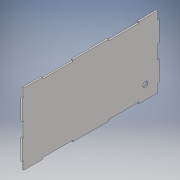
# Autodesk Inventor part: case_side_A
Saved by Autodesk Inventor 2019 (Build 230136000, 136)
## iProperties
Created: 2019-07-12
Part Number: case_side_A
Material: Generic
Document SubType Name: Modeling
Designer: Lino P
Density: 1 g/cm^3
Appearance: Default
Author: Lino P
Autodesk Inventor part; units mm, degrees
ref_plane "YZ Plane" through (0, 0, 0) normal (1, 0, 0) x (0, 1, 0)
ref_plane "XZ Plane" through (0, 0, 0) normal (0, 1, 0) x (-1, 0, 0)
ref_plane "XY Plane" through (0, 0, 0) normal (0, 0, 1) x (1, 0, 0)
sketch "Sketch1" plane through (0, 0, 0) normal (0, 0, 1) x (1, 0, 0)
  line L0 (-15, 60.2) -> (357, 60.2)
  line L1 (357, 60.2) -> (357, -80)
  line L2 (357, -80) -> (-15, -80)
  line L3 (-15, -80) -> (-15, 60.2)
  line L4 (-15, -9.9) -> (357, -9.9) construction
  line L5 (171, 60.2) -> (171, -80) construction
  line L6 (-15, 44.2) -> (-9, 44.2)
  line L7 (-9, 44.2) -> (-9, 4.2)
  line L8 (-9, 4.2) -> (-15, 4.2)
  line L9 (-15, 4.2) -> (-15, 44.2)
  line L10 (-15, -64) -> (-9, -64)
  line L11 (-9, -64) -> (-9, -24)
  line L12 (-9, -24) -> (-15, -24)
  line L13 (-15, -24) -> (-15, -64)
  line L14 (357, 44.2) -> (351, 44.2)
  line L15 (351, 44.2) -> (351, 4.2)
  line L16 (351, 4.2) -> (357, 4.2)
  line L17 (357, 4.2) -> (357, 44.2)
  line L18 (351, -64) -> (351, -24)
  line L19 (357, -64) -> (351, -64)
  line L20 (357, -24) -> (357, -64)
  line L21 (351, -24) -> (357, -24)
  line L22 (25, 60.2) -> (110, 60.2)
  line L23 (110, 60.2) -> (110, 54.2)
  line L24 (110, 54.2) -> (25, 54.2)
  line L25 (25, 54.2) -> (25, 60.2)
  line L26 (317, 60.2) -> (232, 60.2)
  line L27 (232, 60.2) -> (232, 54.2)
  line L28 (232, 54.2) -> (317, 54.2)
  line L29 (317, 54.2) -> (317, 60.2)
  line L30 (25, -80) -> (110, -80)
  line L31 (110, -80) -> (110, -74)
  line L32 (110, -74) -> (25, -74)
  line L33 (25, -74) -> (25, -80)
  line L34 (317, -74) -> (317, -80)
  line L35 (232, -80) -> (232, -74)
  line L36 (232, -74) -> (317, -74)
  line L37 (317, -80) -> (232, -80)
  line L38 (-15, 24.2) -> (357, 24.2) construction
  circle A0 centre (15.4749, 24.2) radius 5
  line L39 (6.5749, 15.3) -> (24.3749, 15.3) construction
  line L40 (24.3749, 15.3) -> (24.3749, 33.1) construction
  line L41 (24.3749, 33.1) -> (6.5749, 33.1) construction
  line L42 (6.5749, 33.1) -> (6.5749, 15.3) construction
  circle A1 centre (9.1249, 30.55) radius 1.05
  line L43 (9.1249, 30.55) -> (9.1249, 31.6) construction
  line L44 (9.1249, 30.55) -> (8.0749, 30.55) construction
  line L45 (15.4749, 33.1) -> (15.4749, 15.3) construction
  line L46 (6.5749, 24.2) -> (24.3749, 24.2) construction
  circle A2 centre (21.8249, 30.55) radius 1.05
  line L47 (21.8249, 30.55) -> (21.8249, 31.6) construction
  line L48 (21.8249, 30.55) -> (22.8749, 30.55) construction
  circle A3 centre (9.1249, 17.85) radius 1.05
  line L49 (9.1249, 17.85) -> (9.1249, 16.8) construction
  line L50 (9.1249, 17.85) -> (8.0749, 17.85) construction
  line L51 (21.8249, 17.85) -> (21.8249, 16.8) construction
  line L52 (21.8249, 17.85) -> (22.8749, 17.85) construction
  circle A4 centre (21.8249, 17.85) radius 1.05
  circle A5 centre (59.8749, 24.2) radius 5
  circle A6 centre (104.2749, 24.2) radius 5
  circle A7 centre (148.6749, 24.2) radius 5
  circle A8 centre (193.0749, 24.2) radius 5
  circle A9 centre (237.4749, 24.2) radius 5
  circle A10 centre (281.8749, 24.2) radius 5
  circle A11 centre (326.2749, 24.2) radius 5
  circle A12 centre (15.4749, -43.8) radius 5
  circle A13 centre (59.8749, -43.8) radius 5
  circle A14 centre (104.2749, -43.8) radius 5
  circle A15 centre (148.6749, -43.8) radius 5
  circle A16 centre (193.0749, -43.8) radius 5
  circle A17 centre (237.4749, -43.8) radius 5
  circle A18 centre (281.8749, -43.8) radius 5
  circle A19 centre (326.2749, -43.8) radius 5
  circle A20 centre (9.1249, -37.45) radius 1.05
  circle A21 centre (21.8249, -37.45) radius 1.05
  circle A22 centre (21.8249, -50.15) radius 1.05
  circle A23 centre (9.1249, -50.15) radius 1.05
  circle A24 centre (53.5249, 30.55) radius 1.05
  circle A25 centre (66.2249, 30.55) radius 1.05
  circle A26 centre (66.2249, 17.85) radius 1.05
  circle A27 centre (53.5249, 17.85) radius 1.05
  circle A28 centre (53.5249, -37.45) radius 1.05
  circle A29 centre (66.2249, -37.45) radius 1.05
  circle A30 centre (66.2249, -50.15) radius 1.05
  circle A31 centre (53.5249, -50.15) radius 1.05
  circle A32 centre (97.9249, 30.55) radius 1.05
  circle A33 centre (110.6249, 30.55) radius 1.05
  circle A34 centre (110.6249, 17.85) radius 1.05
  circle A35 centre (97.9249, 17.85) radius 1.05
  circle A36 centre (97.9249, -37.45) radius 1.05
  circle A37 centre (110.6249, -37.45) radius 1.05
  circle A38 centre (110.6249, -50.15) radius 1.05
  circle A39 centre (97.9249, -50.15) radius 1.05
  circle A40 centre (142.3249, 30.55) radius 1.05
  circle A41 centre (155.0249, 30.55) radius 1.05
  circle A42 centre (155.0249, 17.85) radius 1.05
  circle A43 centre (142.3249, 17.85) radius 1.05
  circle A44 centre (142.3249, -37.45) radius 1.05
  circle A45 centre (155.0249, -37.45) radius 1.05
  circle A46 centre (155.0249, -50.15) radius 1.05
  circle A47 centre (142.3249, -50.15) radius 1.05
  circle A48 centre (186.7249, 30.55) radius 1.05
  circle A49 centre (199.4249, 30.55) radius 1.05
  circle A50 centre (199.4249, 17.85) radius 1.05
  circle A51 centre (186.7249, 17.85) radius 1.05
  circle A52 centre (186.7249, -37.45) radius 1.05
  circle A53 centre (199.4249, -37.45) radius 1.05
  circle A54 centre (199.4249, -50.15) radius 1.05
  circle A55 centre (186.7249, -50.15) radius 1.05
  circle A56 centre (231.1249, 30.55) radius 1.05
  circle A57 centre (243.8249, 30.55) radius 1.05
  circle A58 centre (243.8249, 17.85) radius 1.05
  circle A59 centre (231.1249, 17.85) radius 1.05
  circle A60 centre (231.1249, -37.45) radius 1.05
  circle A61 centre (243.8249, -37.45) radius 1.05
  circle A62 centre (243.8249, -50.15) radius 1.05
  circle A63 centre (231.1249, -50.15) radius 1.05
  circle A64 centre (275.5249, 30.55) radius 1.05
  circle A65 centre (288.2249, 30.55) radius 1.05
  circle A66 centre (288.2249, 17.85) radius 1.05
  circle A67 centre (275.5249, 17.85) radius 1.05
  circle A68 centre (275.5249, -37.45) radius 1.05
  circle A69 centre (288.2249, -37.45) radius 1.05
  circle A70 centre (288.2249, -50.15) radius 1.05
  circle A71 centre (275.5249, -50.15) radius 1.05
  point P0 (0, 0)
  point P1 (9.1249, -36.4)
  point P2 (8.0749, -37.45)
  point P3 (21.8249, -36.4)
  point P4 (22.8749, -37.45)
  point P5 (21.8249, -51.2)
  point P6 (22.8749, -50.15)
  point P7 (9.1249, -51.2)
  point P8 (8.0749, -50.15)
  point P9 (53.5249, 31.6)
  point P10 (52.4749, 30.55)
  point P11 (66.2249, 31.6)
  point P12 (67.2749, 30.55)
  point P13 (66.2249, 16.8)
  point P14 (67.2749, 17.85)
  point P15 (53.5249, 16.8)
  point P16 (52.4749, 17.85)
  point P17 (53.5249, -36.4)
  point P18 (52.4749, -37.45)
  point P19 (66.2249, -36.4)
  point P20 (67.2749, -37.45)
  point P21 (66.2249, -51.2)
  point P22 (67.2749, -50.15)
  point P23 (53.5249, -51.2)
  point P24 (52.4749, -50.15)
  point P25 (97.9249, 31.6)
  point P26 (96.8749, 30.55)
  point P27 (110.6249, 31.6)
  point P28 (111.6749, 30.55)
  point P29 (110.6249, 16.8)
  point P30 (111.6749, 17.85)
  point P31 (97.9249, 16.8)
  point P32 (96.8749, 17.85)
  point P33 (97.9249, -36.4)
  point P34 (96.8749, -37.45)
  point P35 (110.6249, -36.4)
  point P36 (111.6749, -37.45)
  point P37 (110.6249, -51.2)
  point P38 (111.6749, -50.15)
  point P39 (97.9249, -51.2)
  point P40 (96.8749, -50.15)
  point P41 (142.3249, 31.6)
  point P42 (141.2749, 30.55)
  point P43 (155.0249, 31.6)
  point P44 (156.0749, 30.55)
  point P45 (155.0249, 16.8)
  point P46 (156.0749, 17.85)
  point P47 (142.3249, 16.8)
  point P48 (141.2749, 17.85)
  point P49 (142.3249, -36.4)
  point P50 (141.2749, -37.45)
  point P51 (155.0249, -36.4)
  point P52 (156.0749, -37.45)
  point P53 (155.0249, -51.2)
  point P54 (156.0749, -50.15)
  point P55 (142.3249, -51.2)
  point P56 (141.2749, -50.15)
  point P57 (186.7249, 31.6)
  point P58 (185.6749, 30.55)
  point P59 (199.4249, 31.6)
  point P60 (200.4749, 30.55)
  point P61 (199.4249, 16.8)
  point P62 (200.4749, 17.85)
  point P63 (186.7249, 16.8)
  point P64 (185.6749, 17.85)
  point P65 (186.7249, -36.4)
  point P66 (185.6749, -37.45)
  point P67 (199.4249, -36.4)
  point P68 (200.4749, -37.45)
  point P69 (199.4249, -51.2)
  point P70 (200.4749, -50.15)
  point P71 (186.7249, -51.2)
  point P72 (185.6749, -50.15)
  point P73 (231.1249, 31.6)
  point P74 (230.0749, 30.55)
  point P75 (243.8249, 31.6)
  point P76 (244.8749, 30.55)
  point P77 (243.8249, 16.8)
  point P78 (244.8749, 17.85)
  point P79 (231.1249, 16.8)
  point P80 (230.0749, 17.85)
  point P81 (231.1249, -36.4)
  point P82 (230.0749, -37.45)
  point P83 (243.8249, -36.4)
  point P84 (244.8749, -37.45)
  point P85 (243.8249, -51.2)
  point P86 (244.8749, -50.15)
  point P87 (231.1249, -51.2)
  point P88 (230.0749, -50.15)
  point P89 (275.5249, 31.6)
  point P90 (274.4749, 30.55)
  point P91 (288.2249, 31.6)
  point P92 (289.2749, 30.55)
  point P93 (288.2249, 16.8)
  point P94 (289.2749, 17.85)
  point P95 (275.5249, 16.8)
  point P96 (274.4749, 17.85)
  point P97 (275.5249, -36.4)
  point P98 (274.4749, -37.45)
  point P99 (288.2249, -36.4)
  point P100 (289.2749, -37.45)
  point P101 (288.2249, -51.2)
  point P102 (289.2749, -50.15)
  point P103 (275.5249, -51.2)
  point P104 (274.4749, -50.15)
  dimension "d38" = 6
  dimension "d41" = 6
  dimension "d42" = 40
  dimension "d43" = 85
  dimension "d46" = 10
  dimension "d47" = 17.8
  dimension "d48" = 17.8
  dimension "d50" = 1.5
  dimension "d51" = 2.1
  dimension "d52" = 1.5
  dimension "d55" = 44.4
  dimension "d58" = 68
  dimension "d63" = 68
  dimension "d66" = 44.4
  constraints: 112 point on circle, 106 end point, 72 centre point, 33 symmetric about line, 9 midpoint, 8 parallel, 6 horizontal, 5 perpendicular, 3 point on line, 3 vertical, 241 other
  measures "d38" distance of L7.end L8.end
  measures "d41" distance of L22.end L23.end
  measures "d42" distance between parallel lines of L25 L3
  measures "d43" distance between parallel lines of L25 L23
  measures "d46" diameter of A0
  measures "d47" distance of L41.end L40.end
  measures "d48" distance of L40.end L39.end
  measures "d50" distance from line of L42 L44.end
  measures "d51" diameter of A1
  measures "d52" distance from line of L41 L43.end
  measures "d55" distance of A0.centre A5.centre
  measures "d58" distance of A0.centre A12.centre
  measures "d63" distance of L43.start A20.centre
  measures "d66" distance of L43.start A24.centre
ref_plane "Work Plane1" through (351, 4.2, 0) normal (1, 0, 0) x (0, 0, -1)
sketch "Sketch2" plane through (351, 4.2, 0) normal (1, 0, 0) x (0, 0, -1)
  line L0 (0, 40) -> (0, 0) projected
  line L1 (0, 40) -> (-6, 40) projected
  line L2 (-6, 0) -> (-6, 40) projected
  line L3 (0, 0) -> (-6, 0) projected
  line L4 (-6, 40) -> (0, 40) projected
  line L5 (0, 40) -> (0, 56) projected
  line L6 (0, 56) -> (-6, 56) projected
  line L7 (-6, 40) -> (-6, 56) projected
  line L8 (-6, -28.2) -> (0, -28.2) projected
  line L9 (0, -28.2) -> (0, 0) projected
  line L10 (0, 0) -> (-6, 0) projected
  line L11 (-6, -28.2) -> (-6, 0) projected
  line L12 (0, -28.2) -> (0, -68.2) projected
  line L13 (0, -28.2) -> (-6, -28.2) projected
  line L14 (-6, -68.2) -> (-6, -28.2) projected
  line L15 (0, -68.2) -> (-6, -68.2) projected
  line L16 (0, -68.2) -> (-6, -68.2) projected
  line L17 (-6, -84.2) -> (-6, -68.2) projected
  line L18 (0, -84.2) -> (-6, -84.2) projected
  line L19 (0, -84.2) -> (0, -68.2) projected
  line L20 (-6, 56) -> (264, 56)
  line L21 (264, 56) -> (264, -84.2)
  line L22 (264, -84.2) -> (-6, -84.2)
  line L23 (-6, -84.2) -> (-6, 56)
  line L24 (129, 56) -> (129, -84.2) construction
  line L25 (258, 40) -> (258, 0)
  line L26 (258, 40) -> (264, 40)
  line L27 (264, 0) -> (264, 40)
  line L28 (258, 0) -> (264, 0)
  line L29 (264, 40) -> (258, 40)
  line L30 (258, 40) -> (258, 56)
  line L31 (258, 56) -> (264, 56)
  line L32 (264, 40) -> (264, 56)
  line L33 (264, -28.2) -> (258, -28.2)
  line L34 (258, -28.2) -> (258, 0)
  line L35 (258, 0) -> (264, 0)
  line L36 (264, -28.2) -> (264, 0)
  line L37 (258, -28.2) -> (258, -68.2)
  line L38 (258, -28.2) -> (264, -28.2)
  line L39 (264, -68.2) -> (264, -28.2)
  line L40 (258, -68.2) -> (264, -68.2)
  line L41 (258, -68.2) -> (264, -68.2)
  line L42 (264, -84.2) -> (264, -68.2)
  line L43 (258, -84.2) -> (264, -84.2)
  line L44 (258, -84.2) -> (258, -68.2)
  line L45 (264, -84.2) -> (264, 56)
  line L46 (34, 56) -> (94, 56)
  line L47 (94, 56) -> (94, 53)
  line L48 (94, 53) -> (34, 53)
  line L49 (34, 53) -> (34, 56)
  line L50 (224, 56) -> (164, 56)
  line L51 (164, 56) -> (164, 53)
  line L52 (164, 53) -> (224, 53)
  line L53 (224, 53) -> (224, 56)
  line L54 (-6, -14.1) -> (264, -14.1) construction
  line L55 (34, -84.2) -> (94, -84.2)
  line L56 (94, -84.2) -> (94, -81.2)
  line L57 (94, -81.2) -> (34, -81.2)
  line L58 (34, -81.2) -> (34, -84.2)
  line L59 (164, -84.2) -> (164, -81.2)
  line L60 (164, -81.2) -> (224, -81.2)
  line L61 (224, -84.2) -> (164, -84.2)
  line L62 (224, -81.2) -> (224, -84.2)
  point P0 (0, -4.2)
  point P1 (258, -4.2)
  dimension "d71" = 270
  dimension "d72" = 60
  dimension "d73" = 3
  dimension "d74" = 40
  constraints: 86 end point, 33 symmetric about line, 4 midpoint, 4 parallel, 2 horizontal, 2 perpendicular, 1 point on line
  measures "d71" distance of L21.end L22.end
  measures "d72" distance of L47.end L48.end
  measures "d73" distance of L46.end L47.end
  measures "d74" distance between parallel lines of L2 L49
extrude "Extrusion3" add sketch "Sketch2" along normal blind 3 contours L5 L20 L49 L48 L47 L51 L52 L53 L30 L25 L34 L37 L44 L22 L62 L60 L59 L56 L57 L58 L19 L12 L9 L0 | L0 L3 L2 L1 | L12 L15 L14 L8 | L26 L21 L28 L25 | L33 L21 L40 L37
sketch "Sketch3" plane through (354, 4.2, 0) normal (1, 0, 0) x (0, 0, -1)
  line L0 (164, -84.2) -> (164, -81.2) construction
  line L1 (164, -81.2) -> (224, -81.2) construction
  line L2 (224, -81.2) -> (224, -84.2) construction
  line L3 (224, -84.2) -> (258, -84.2) construction
  line L4 (258, -84.2) -> (258, -68.2) construction
  line L5 (258, -68.2) -> (264, -68.2) construction
  line L6 (264, -68.2) -> (264, -28.2) construction
  line L7 (264, -28.2) -> (258, -28.2) construction
  line L8 (258, -28.2) -> (258, 0) construction
  line L9 (258, 0) -> (264, 0) construction
  line L10 (264, 0) -> (264, 40) construction
  line L11 (264, 40) -> (258, 40) construction
  line L12 (258, 40) -> (258, 56) construction
  line L13 (258, 56) -> (224, 56) construction
  line L14 (224, 56) -> (224, 53) construction
  line L15 (224, 53) -> (164, 53) construction
  line L16 (164, 53) -> (164, 56) construction
  line L17 (164, 56) -> (94, 56) construction
  line L18 (94, 56) -> (94, 53) construction
  line L19 (94, 53) -> (34, 53) construction
  line L20 (34, 53) -> (34, 56) construction
  line L21 (34, 56) -> (0, 56) construction
  line L22 (0, 56) -> (0, 40) construction
  line L23 (0, 40) -> (-6, 40) construction
  line L24 (-6, 40) -> (-6, 0) construction
  line L25 (-6, 0) -> (0, 0) construction
  line L26 (0, 0) -> (0, -28.2) construction
  line L27 (0, -28.2) -> (-6, -28.2) construction
  line L28 (-6, -28.2) -> (-6, -68.2) construction
  line L29 (-6, -68.2) -> (0, -68.2) construction
  line L30 (0, -68.2) -> (0, -84.2) construction
  line L31 (0, -84.2) -> (34, -84.2) construction
  line L32 (34, -84.2) -> (34, -81.2) construction
  line L33 (34, -81.2) -> (94, -81.2) construction
  line L34 (94, -81.2) -> (94, -84.2) construction
  line L35 (94, -84.2) -> (164, -84.2) construction
  circle A0 centre (236.3286, -56.9983) radius 5
  point P0 (0, -4.2)
  dimension "d77" = 10
  constraints: 1 centre point
  measures "d77" diameter of A0
extrude "Extrusion4" cut sketch "Sketch3" against normal blind 10
sketch "Sketch4" plane through (354, 4.2, 0) normal (1, 0, 0) x (0, 0, -1)
  circle A0 centre (236.3286, -56.9983) radius 5 construction
  line L0 (164, -84.2) -> (164, -81.2) construction
  line L1 (164, -81.2) -> (224, -81.2) construction
  line L2 (224, -81.2) -> (224, -84.2) construction
  line L3 (224, -84.2) -> (258, -84.2) construction
  line L4 (258, -84.2) -> (258, -68.2) construction
  line L5 (258, -68.2) -> (264, -68.2) construction
  line L6 (264, -68.2) -> (264, -28.2) construction
  line L7 (264, -28.2) -> (258, -28.2) construction
  line L8 (258, -28.2) -> (258, 0) construction
  line L9 (258, 0) -> (264, 0) construction
  line L10 (264, 0) -> (264, 40) construction
  line L11 (264, 40) -> (258, 40) construction
  line L12 (258, 40) -> (258, 56) construction
  line L13 (258, 56) -> (224, 56) construction
  line L14 (224, 56) -> (224, 53) construction
  line L15 (224, 53) -> (164, 53) construction
  line L16 (164, 53) -> (164, 56) construction
  line L17 (164, 56) -> (94, 56) construction
  line L18 (94, 56) -> (94, 53) construction
  line L19 (94, 53) -> (34, 53) construction
  line L20 (34, 53) -> (34, 56) construction
  line L21 (34, 56) -> (0, 56) construction
  line L22 (0, 56) -> (0, 40) construction
  line L23 (0, 40) -> (-6, 40) construction
  line L24 (-6, 40) -> (-6, 0) construction
  line L25 (-6, 0) -> (0, 0) construction
  line L26 (0, 0) -> (0, -28.2) construction
  line L27 (0, -28.2) -> (-6, -28.2) construction
  line L28 (-6, -28.2) -> (-6, -68.2) construction
  line L29 (-6, -68.2) -> (0, -68.2) construction
  line L30 (0, -68.2) -> (0, -84.2) construction
  line L31 (0, -84.2) -> (34, -84.2) construction
  line L32 (34, -84.2) -> (34, -81.2) construction
  line L33 (34, -81.2) -> (94, -81.2) construction
  line L34 (94, -81.2) -> (94, -84.2) construction
  line L35 (94, -84.2) -> (164, -84.2) construction
  line L36 (0, 56) -> (-3, 56)
  line L37 (-3, 56) -> (-3, -84.2)
  line L38 (-3, -84.2) -> (0, -84.2)
  line L39 (0, -84.2) -> (0, 56)
  line L40 (164, 56) -> (94, 56) construction
  line L41 (129, 56) -> (129, -84.2) construction
  line L42 (258, 56) -> (258, 40) construction
  line L43 (258, 40) -> (264, 40) construction
  line L44 (264, 40) -> (264, 0) construction
  line L45 (264, 0) -> (258, 0) construction
  line L46 (258, 0) -> (258, -28.2) construction
  line L47 (258, -28.2) -> (264, -28.2) construction
  line L48 (264, -28.2) -> (264, -68.2) construction
  line L49 (264, -68.2) -> (258, -68.2) construction
  line L50 (258, -68.2) -> (258, -84.2) construction
  line L51 (258, 56) -> (261, 56)
  line L52 (261, 56) -> (261, -84.2)
  line L53 (261, -84.2) -> (258, -84.2)
  line L54 (258, -84.2) -> (258, 56)
  point P0 (0, -4.2)
  point P1 (258, -4.2)
  dimension "d80" = 3
  constraints: 36 end point, 5 symmetric about line, 2 midpoint, 2 parallel, 1 horizontal, 1 perpendicular
  measures "d80" distance of L38.end L37.end
extrude "Extrusion5" add sketch "Sketch4" against normal blind 3
body "Solid1"
